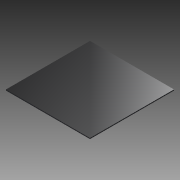
# Autodesk Inventor part: EnclosurePanelSide
Saved by Autodesk Inventor 2015 SP1 (Build 190203100, 203)
## iProperties
Created: 2015-01-12
Part Number: EnclosurePanelSide
Material: ABS Plastic
Document SubType Name: Modeling
Designer: Jack
Density: 1.06 g/cm^3
Appearance: Smooth - Dark Gray
Mass: 595.148 g
Surface Area: 2867.62 cm^2
Volume: 561.46 cm^3
Author: Jack
Autodesk Inventor part; units mm, degrees
ref_plane "YZ Plane" through (0, 0, 0) normal (1, 0, 0) x (0, 1, 0)
ref_plane "XZ Plane" through (0, 0, 0) normal (0, 1, 0) x (-1, 0, 0)
ref_plane "XY Plane" through (0, 0, 0) normal (0, 0, 1) x (1, 0, 0)
sketch "Sketch1" plane through (0, 0, 0) normal (0, 0, 1) x (1, 0, 0)
  line L0 (0, 0) -> (419.7625, 0)
  line L1 (419.7625, 0) -> (419.7625, 420)
  line L2 (419.7625, 420) -> (0, 420)
  line L3 (0, 420) -> (0, 0)
  dimension "d0" = 419.7625
  dimension "d1" = 420
  constraints: 8 end point, 2 parallel, 1 horizontal, 1 perpendicular
  measures "d0" distance of L2.end L1.end
  measures "d1" distance of L0.end L1.end
extrude "Extrusion1" add sketch "Sketch1" along normal blind 4.7625
sketch "Sketch3" plane through (0, 0, 4.7625) normal (0, 0, 1) x (1, 0, 0)
  line L0 (0, 0) -> (419.7625, 0) projected
  line L1 (419.7625, 0) -> (419.7625, 420) projected
  line L2 (0, 420) -> (0, 0) projected
  circle A0 centre (130, 40) radius 19.05
  circle A1 centre (289.7625, 40) radius 19.05
  dimension "d13" = 38.1
  dimension "d14" = 130
  dimension "d15" = 130
  dimension "d16" = 40
  constraints: 2 centre point, 1 equal radius, 1 horizontal alignment
  measures "d13" diameter of A0
  measures "d14" distance from line of L2 A0.centre
  measures "d15" distance from line of L1 A1.centre
  measures "d16" distance from line of L0 A1.centre
extrude "Extrusion2" cut sketch "Sketch3" against normal up to next
sketch "Sketch4" plane through (0, 0, 4.7625) normal (0, 0, 1) x (1, 0, 0)
  circle A0 centre (130, 40) radius 19.05 projected
  circle A1 centre (289.7625, 40) radius 19.05 projected
  point P0 (114, 56)
  point P1 (146, 56)
  point P2 (114, 24)
  point P3 (146, 24)
  point P4 (273.7625, 56)
  point P5 (305.7625, 56)
  point P6 (273.7625, 24)
  point P7 (305.7625, 24)
  dimension "d11" = 32
  dimension "d12" = 32
  dimension "d17" = 16
  dimension "d18" = 16
  dimension "d19" = 32
  dimension "d20" = 32
  dimension "d21" = 16
  dimension "d22" = 16
  constraints: 4 horizontal alignment, 4 vertical alignment
  measures "d11" distance of point (146, 56) point (114, 56)
  measures "d12" distance of point (114, 56) point (114, 24)
  measures "d17" horizontal distance of A0.centre point (114, 56)
  measures "d18" horizontal distance of point (146, 56) A0.centre
  measures "d19" distance of point (305.762, 56) point (273.762, 56)
  measures "d20" distance of point (273.762, 56) point (273.762, 24)
  measures "d21" horizontal distance of A1.centre point (273.762, 56)
  measures "d22" horizontal distance of point (305.762, 56) A1.centre
hole "Hole1" at (114, 56, 4.7625) at (146, 56, 4.7625) at (114, 24, 4.7625) at (146, 24, 4.7625) at (273.7625, 56, 4.7625) at (305.7625, 56, 4.7625) at (273.7625, 24, 4.7625) at (305.7625, 24, 4.7625) direction (0, 0, -1) diameter 3.5 end through all
body "Solid1"
